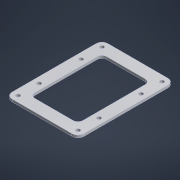
# Autodesk Inventor part: P018
Saved by Autodesk Inventor 2021.3 (Build 253353000, 353)
## iProperties
Company: HES-SO
Created: 2022-05-28
Part Number: P018
Material: Polytetrafluoroethylene
Document SubType Name: Modeling
Designer: HER & ZAE
Density: 2.02 g/cm^3
Appearance: PTFE
Mass: 9.39799 g
Surface Area: 57.4453 cm^2
Volume: 4.65247 cm^3
Author: HER & ZAE
Title: Joint Carter Chapeau
Autodesk Inventor part; units mm, degrees
ref_plane "YZ Plane" through (0, 0, 0) normal (1, 0, 0) x (0, 1, 0)
ref_plane "XZ Plane" through (0, 0, 0) normal (0, 1, 0) x (-1, 0, 0)
ref_plane "XY Plane" through (0, 0, 0) normal (0, 0, 1) x (1, 0, 0)
sketch "Sketch2" plane through (0, 0, 0) normal (0, 0, 1) x (1, 0, 0)
  arc A0 (-30, -45) -> (-25, -50) centre (-25, -45) ccw projected
  line L0 (-25, -50) -> (25, -50) projected
  arc A1 (25, -50) -> (30, -45) centre (25, -45) ccw projected
  line L1 (30, -45) -> (30, 25) projected
  arc A2 (30, 25) -> (25, 30) centre (25, 25) ccw projected
  line L2 (25, 30) -> (-25, 30) projected
  arc A3 (-25, 30) -> (-30, 25) centre (-25, 25) ccw projected
  line L3 (-30, 25) -> (-30, -45) projected
  circle A4 centre (25, -27.5) radius 1.621 projected
  circle A5 centre (-25, 7.5) radius 1.621 projected
  circle A6 centre (-25, 25) radius 1.621 projected
  circle A7 centre (25, -45) radius 1.621 projected
  circle A8 centre (-25, -45) radius 1.621 projected
  circle A9 centre (25, 25) radius 1.621 projected
  circle A10 centre (-25, -27.5) radius 1.621 projected
  circle A11 centre (25, 7.5) radius 1.621 projected
  line L4 (16, -40) -> (-16, -40) projected
  arc A12 (-20, -36) -> (-16, -40) centre (-16, -36) ccw projected
  line L5 (-20, -36) -> (-20, 16) projected
  arc A13 (-16, 20) -> (-20, 16) centre (-16, 16) ccw projected
  line L6 (-16, 20) -> (16, 20) projected
  arc A14 (20, 16) -> (16, 20) centre (16, 16) ccw projected
  line L7 (20, 16) -> (20, -36) projected
  arc A15 (16, -40) -> (20, -36) centre (16, -36) ccw projected
extrude "Extrusion1" add sketch "Sketch2" against normal blind 2
body "Solid1"
